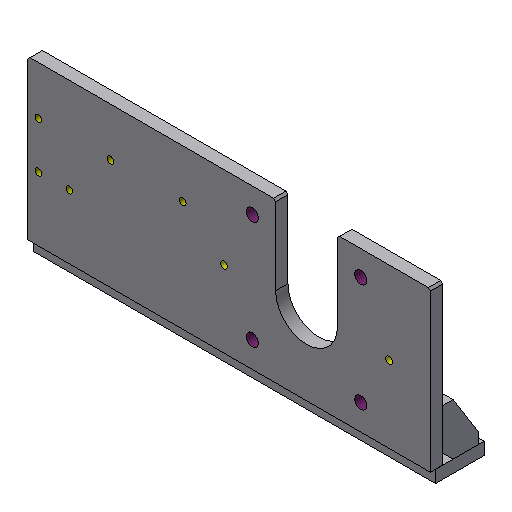
# Autodesk Inventor part: TL20240701-10110CV-005
Saved by Autodesk Inventor 2022.5 (Build 265521000, 521)
## iProperties
Category: DRIVE UNIT ASSY
Company: 현대 트랜시스(대유)
Created: 2023-04-10
Part Number: TL20240701-10110CV-005
Checked By: 김형민
Engr Approved By: 김시현
User Status: 1/1 x18
Material: SS400
Description: 0
Document SubType Name: Modeling
Mfg Approved By: 호상태
Designer: 박성규
Stock Number: 005
Density: 7.85 g/cm^3
Appearance: Painting-RAL7035
Project: SW PJT
DETAIL: Coveryor Assembly
M/C TITLE: CJ 제일제당 협동로봇 포장시스탬 PILOT 장비
PARTS NAME: Bracket
SPECIFICATION: TA20221101-CV200000-015
DocNumber: 221118_Standard_v1
Folder: .\
VDS_Category: 엔지니어링
Title: PLATE
Subject: SW차종 시트조립라인
Author: 박성규
Revision Number: A
Autodesk Inventor part; units mm, degrees
ref_plane "YZ Plane" through (0, 0, 0) normal (1, 0, 0) x (0, 1, 0)
ref_plane "XZ Plane" through (0, 0, 0) normal (0, 1, 0) x (-1, 0, 0)
ref_plane "XY Plane" through (0, 0, 0) normal (0, 0, 1) x (1, 0, 0)
sketch "스케치9" plane through (0, 0, 0) normal (0, 0, 1) x (1, 0, 0)
  line L0 (-195, 77) -> (195, 77)
  line L1 (195, 77) -> (195, -77)
  line L2 (195, -77) -> (-195, -77)
  line L3 (-195, -77) -> (-195, 77)
  line L4 (-195, 77) -> (195, -77) construction
  line L5 (195, 77) -> (-195, -77) construction
  point P0 (0, 0)
  dimension "d40" = 390
  dimension "d41" = 154
  constraints: 12 end point, 2 midpoint, 2 parallel, 1 horizontal, 1 perpendicular
  measures "d40" distance of L0.start L0.end
  measures "d41" distance of L0.end L1.end
extrude "돌출4" add sketch "스케치9" along normal mid plane 12
sketch "스케치10" plane through (195, -77, 6) normal (1, 0, 0) x (0, 0, -1)
  line L0 (0, 0) -> (0, 154) construction
  line L1 (12, 0) -> (0, 0) construction
  line L2 (5, 0) -> (52, 0)
  line L3 (52, 0) -> (52, -12)
  line L4 (52, -12) -> (5, -12)
  line L5 (5, -12) -> (5, 0)
  line L6 (12, 154) -> (12, 0) construction
  point P0 (6, 77)
  dimension "d44" = 47
  dimension "d45" = 12
  dimension "d46" = 5
  dimension "d47" = 52
  dimension "d50" = 40
  constraints: 8 end point, 2 parallel, 1 horizontal, 1 perpendicular, 1 point on line
  measures "d44" distance of L3.end L4.end
  measures "d45" distance of L4.end L2.start
  measures "d46" distance between parallel lines of L0 L5
  measures "d47" distance between parallel lines of L3 L0
  measures "d50" distance between parallel lines of L6 L3
extrude "돌출5" add sketch "스케치10" against normal up to surface (390 mm away) separate body
sketch "스케치11" plane through (195, -77, 1) normal (0, 1, 0) x (1, 0, 0)
  line L0 (0, 47) -> (-390, 47) construction
  line L1 (-360, 39) -> (-360, 25) construction
  line L2 (-365.5, 39) -> (-365.5, 25)
  line L3 (-354.5, 25) -> (-354.5, 39)
  arc A0 (-354.5, 39) -> (-365.5, 39) centre (-360, 39) ccw
  arc A1 (-365.5, 25) -> (-354.5, 25) centre (-360, 25) ccw
  line L4 (-195, 39) -> (-195, 25) construction
  line L5 (-200.5, 39) -> (-200.5, 25)
  line L6 (-189.5, 25) -> (-189.5, 39)
  arc A2 (-189.5, 39) -> (-200.5, 39) centre (-195, 39) ccw
  arc A3 (-200.5, 25) -> (-189.5, 25) centre (-195, 25) ccw
  line L7 (-30, 39) -> (-30, 25) construction
  line L8 (-35.5, 39) -> (-35.5, 25)
  line L9 (-24.5, 25) -> (-24.5, 39)
  arc A4 (-24.5, 39) -> (-35.5, 39) centre (-30, 39) ccw
  arc A5 (-35.5, 25) -> (-24.5, 25) centre (-30, 25) ccw
  line L10 (-390, 47) -> (-390, 0) projected
  point P0 (-195, 1)
  point P1 (-30, 32)
  point P2 (-195, 32)
  point P3 (-360, 32)
  point P4 (-360, 44.5)
  point P5 (-195, 44.5)
  point P6 (-30, 44.5)
  dimension "d51" = 15
  dimension "d53" = 165
  dimension "d54" = 165
  dimension "d122" = 11
  dimension "d123" = 12.5
  dimension "d124" = 11
  dimension "d125" = 12.5
  dimension "d126" = 11
  dimension "d127" = 12.5
  dimension "d130" = 30
  constraints: 24 end point, 15 point on circle, 12 tangent, 6 centre point, 3 midpoint, 3 parallel, 3 vertical, 2 horizontal alignment
  measures "d51" distance from line of L0 point (-30, 32)
  measures "d53" distance of point (-195, 32) point (-30, 32)
  measures "d54" distance of point (-360, 32) point (-195, 32)
  measures "d122" diameter of A1
  measures "d123" distance of point (-360, 44.5) point (-360, 32)
  measures "d124" distance between parallel lines of L6 L5
  measures "d125" distance of point (-195, 44.5) point (-195, 32)
  measures "d126" distance between parallel lines of L9 L8
  measures "d127" distance of point (-30, 44.5) point (-30, 32)
  measures "d130" distance between parallel lines of L1 L10
sketch "스케치12" plane through (0, 0, -6) normal (0, 0, -1) x (-1, 0, 0)
  line L0 (195, 77) -> (-195, 77) construction
  line L1 (-195, 77) -> (-195, -77) construction
  line L2 (-75, 0.35) -> (-75, 77) construction
  line L3 (-45, 0.35) -> (-45, 77)
  line L4 (-105, 77) -> (-105, 0.35)
  arc A0 (-105, 0.35) -> (-45, 0.35) centre (-75, 0.35) ccw
  arc A1 (-45, 77) -> (-105, 77) centre (-75, 77) ccw
  point P0 (0, 0)
  point P1 (-75, 38.675)
  dimension "d62" = 76.65
  dimension "d63" = 120
  dimension "d65" = 60
  constraints: 8 end point, 4 point on circle, 4 tangent, 2 centre point, 1 midpoint, 1 parallel, 1 point on line, 1 vertical
  measures "d62" distance from line of L0 L2.start
  measures "d63" distance between parallel lines of L1 L2
  measures "d65" distance between parallel lines of L3 L4
extrude "돌출6" cut sketch "스케치12" against normal through all bodies 1
sketch "스케치13" plane through (0, 0, -6) normal (0, 0, -1) x (-1, 0, 0)
  arc A0 (-105, 0.35) -> (-45, 0.35) centre (-75, 0.35) ccw construction
  line L0 (-127.5, -52.15) -> (-22.5, -52.15)
  line L1 (-22.5, -52.15) -> (-22.5, 52.85)
  line L2 (-22.5, 52.85) -> (-127.5, 52.85)
  line L3 (-127.5, 52.85) -> (-127.5, -52.15)
  line L4 (-127.5, -52.15) -> (-22.5, 52.85) construction
  line L5 (-22.5, -52.15) -> (-127.5, 52.85) construction
  point P0 (0, 0)
  dimension "d68" = 105
  dimension "d69" = 105
  constraints: 12 end point, 4 coincident, 2 midpoint, 2 parallel, 1 horizontal, 1 perpendicular
  measures "d68" distance of L1.end L2.end
  measures "d69" distance of L0.end L1.end
hole "구멍4" at (127.5, 52.85, -6) at (22.5, 52.85, -6) at (22.5, -52.15, -6) at (127.5, -52.15, -6) direction (0, 0, 1) diameter 11.835 end through all bodies 1 thread size "M14x2" class "6H" standard "ISO Metric profile"
sketch "스케치14" plane through (0, 0, -6) normal (0, 0, -1) x (-1, 0, 0)
  line L0 (195, -77) -> (195, 77) construction
  line L1 (195, 77) -> (-45, 77) construction
  point P0 (0, 0)
  point P1 (185, 30)
  point P2 (115, 30)
  point P3 (45, 30)
  point P4 (185, -15)
  point P5 (155, -15)
  dimension "d77" = 30
  dimension "d78" = 10
  dimension "d79" = 10
  dimension "d80" = 92
  dimension "d81" = 47
  dimension "d82" = 70
  dimension "d83" = 70
  constraints: 3 horizontal alignment
  measures "d77" distance of point (185, -15) point (155, -15)
  measures "d78" distance from line of L0 point (185, 30)
  measures "d79" distance from line of L0 point (185, -15)
  measures "d80" distance from line of L1 point (185, -15)
  measures "d81" distance from line of L1 point (185, 30)
  measures "d82" distance of point (185, 30) point (115, 30)
  measures "d83" distance of point (115, 30) point (45, 30)
hole "구멍5" at (-185, 30, -6) at (-115, 30, -6) at (-45, 30, -6) at (-185, -15, -6) at (-155, -15, -6) direction (0, 0, 1) diameter 6.6 end through all bodies 1 clearance for "Socket Head Cap Screw ISO 4762" size "M6" standard "ISO"
sketch "스케치15" plane through (195, -77, 6) normal (1, 0, 0) x (0, 0, -1)
  line L0 (12, 0) -> (0, 0) construction
  line L1 (22, 0) -> (47, 0)
  line L2 (47, 0) -> (47, 10)
  line L3 (22, 50) -> (12, 50)
  line L4 (12, 50) -> (12, 10)
  line L5 (12, 10) -> (22, 0)
  line L6 (22, 50) -> (47, 10)
  point P0 (6, 77)
  point P1 (47, 50)
  dimension "d91" = 50
  dimension "d92" = 35
  dimension "d93" = 10
  dimension "d94" = 10
  dimension "d95" = 25
  dimension "d96" = 40
  constraints: 12 end point, 4 point on line, 2 parallel, 1 horizontal, 1 perpendicular
  measures "d91" distance of L1.end point (47, 50)
  measures "d92" distance of point (47, 50) L3.end
  measures "d93" distance of L4.end L0.start
  measures "d94" distance of L1.start L0.start
  measures "d95" distance of L3.start point (47, 50)
  measures "d96" distance of L2.end point (47, 50)
extrude "돌출7" add sketch "스케치15" against normal blind 9 separate body
mirror "미러1" about plane through (0, 0, 0) normal (1, 0, 0) of "돌출7" bodies 3
chamfer "모따기1" distance 2 angle 45 4 edges at (105, 77, 0) (45, 77, 0) (195, 77, 0) (-195, 77, 0)
sketch "스케치16" plane through (0, 0, -6) normal (0, 0, -1) x (-1, 0, 0)
  line L0 (195, -77) -> (195, 75) construction
  line L1 (-195, -89) -> (195, -89) construction
  point P0 (0, 0)
  point P1 (135, -42)
  point P2 (115, -42)
  dimension "d102" = 60
  dimension "d103" = 47
  dimension "d104" = 20
  constraints: 1 horizontal alignment
  measures "d102" distance from line of L0 point (135, -42)
  measures "d103" distance from line of L1 point (135, -42)
  measures "d104" distance of point (135, -42) point (115, -42)
hole "구멍6" [suppressed]
sketch "스케치17" plane through (0, 0, -6) normal (0, 0, -1) x (-1, 0, 0)
  line L0 (-107, 77) -> (-193, 77) construction
  line L1 (-195, 75) -> (-195, -77) construction
  point P0 (0, 0)
  point P1 (-155, -3)
  point P2 (5, -3)
  dimension "d112" = 40
  dimension "d113" = 80
  dimension "d114" = 160
  constraints: 1 horizontal alignment
  measures "d112" distance from line of L1 point (-155, -3)
  measures "d113" distance from line of L0 point (-155, -3)
  measures "d114" distance of point (-155, -3) point (5, -3)
hole "구멍7" at (155, -3, -6) at (-5, -3, -6) direction (0, 0, 1) diameter 6.6 end through all bodies 1 clearance for "Countersunk Flat Head Screw ISO 2009/7046" size "M6" standard "ISO"
extrude "돌출8" cut sketch "스케치11" against normal through all bodies 2
sketch "스케치18" plane through (195, -77, 1) normal (0, 1, 0) x (1, 0, 0)
  arc A0 (-354.5, 39) -> (-365.5, 39) centre (-360, 39) ccw projected
  arc A1 (-365.5, 25) -> (-354.5, 25) centre (-360, 25) ccw projected
  line L0 (-360, 39) -> (-360, 25)
  arc A2 (-189.5, 39) -> (-200.5, 39) centre (-195, 39) ccw projected
  arc A3 (-200.5, 25) -> (-189.5, 25) centre (-195, 25) ccw projected
  line L1 (-195, 39) -> (-195, 25)
  arc A4 (-24.5, 39) -> (-35.5, 39) centre (-30, 39) ccw projected
  arc A5 (-35.5, 25) -> (-24.5, 25) centre (-30, 25) ccw projected
  line L2 (-30, 39) -> (-30, 25)
  point P0 (-195, 1)
  point P1 (-360, 32)
  point P2 (-195, 32)
  point P3 (-30, 32)
  constraints: 6 end point, 3 midpoint, 3 vertical
equation "\"d54\" = d53"
equation "\"d123\" = d125"
equation "\"d127\" = d125"
equation "\"d83\" = d82"
equation "\"d94\" = d93"
